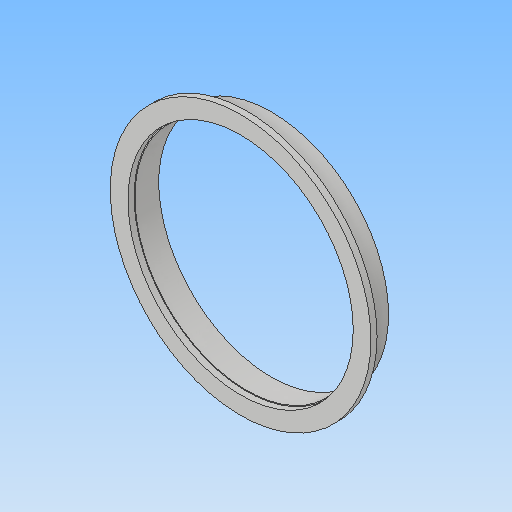
# Autodesk Inventor part: 20_Lens_holder_156mm_clamp
Saved by Autodesk Inventor 2019.4 (Build 234330000, 330)
## iProperties
Created: 2019-10-23
Part Number: 20_Lens_holder_156mm_clamp
Material: Generic
Document SubType Name: Modeling
Designer: marsikovabarbora
Density: 1 g/cm^3
Appearance: Default
Author: marsikovabarbora
Autodesk Inventor part; units mm, degrees
ref_plane "YZ Plane" through (0, 0, 0) normal (1, 0, 0) x (0, 1, 0)
ref_plane "XZ Plane" through (0, 0, 0) normal (0, 1, 0) x (-1, 0, 0)
sketch "Sketch1" plane through (0, 0, 0) normal (0, 0, 1) x (1, 0, 0)
  line L0 (16.8, 24.9006) -> (-16.8, 24.9006) projected
  line L1 (-16.8, 24.9006) -> (-16.8, 21.2406) projected
  line L2 (-16.8, 21.2406) -> (-21.2406, 16.8) projected
  line L3 (-21.2406, 16.8) -> (-24.9006, 16.8) projected
  line L4 (-24.9006, 16.8) -> (-24.9006, -16.8) projected
  line L5 (-24.9006, -16.8) -> (-21.2406, -16.8) projected
  line L6 (-21.2406, -16.8) -> (-16.8, -21.2406) projected
  line L7 (-16.8, -21.2406) -> (-16.8, -24.9006) projected
  line L8 (-16.8, -24.9006) -> (16.8, -24.9006) projected
  line L9 (16.8, -24.9006) -> (16.8, -21.2406) projected
  line L10 (16.8, -21.2406) -> (21.2406, -16.8) projected
  line L11 (21.2406, -16.8) -> (24.9006, -16.8) projected
  line L12 (24.9006, -16.8) -> (24.9006, 16.8) projected
  line L13 (24.9006, 16.8) -> (21.2406, 16.8) projected
  line L14 (21.2406, 16.8) -> (16.8, 21.2406) projected
  line L15 (16.8, 21.2406) -> (16.8, 24.9006) projected
  arc A0 (-24.9006, -4.1858) -> (-4.1858, -24.9006) centre (0, 0) ccw
  circle A1 centre (0, 0) radius 19.1
  circle A2 centre (0, 0) radius 18.1
  circle A3 centre (0, 0) radius 20.6
  circle A4 centre (0, 0) radius 19.6 construction
  circle A5 centre (0, 0) radius 20.6 construction
  circle A6 centre (0, 0) radius 20.6 construction
  point P0 (0, 0)
  dimension "d14" = 38.2
  dimension "d17" = 1
  constraints: 7 centre point, 2 point on circle, 1 coincident, 12 other
  measures "d14" diameter of A1
  measures "d17" radial gap between concentric circles of A1 A2
ref_plane "Work Plane1" through (-13.5, -13.5, -4) normal (0, 0, 1) x (1, 0, 0)
extrude "Extrusion1" add sketch "Sketch1" against normal blind 4 draft -2 contours A1
sketch "Sketch2" plane through (0, 0, 0) normal (0, 0, 1) x (1, 0, 0)
  line L0 (0, -33.742) -> (0, 37.252) construction
  arc A0 (2, 25.1004) -> (-2, 25.1004) centre (0, 25.11) ccw
  circle A1 centre (0, 0) radius 19.1 projected
  circle A2 centre (0, 0) radius 21.1
  circle A3 centre (0, 0) radius 18.2397 projected
  point P0 (0, 0)
  dimension "d5" = 2
  dimension "d16" = 2
  constraints: 2 centre point, 2 point on circle, 1 point on line
  measures "d5" radius of A0
  measures "d16" radial gap between concentric circles of A1 A2
extrude "Extrusion2" add sketch "Sketch2" along normal blind 1 contours A1 | A2
body "Solid1"
